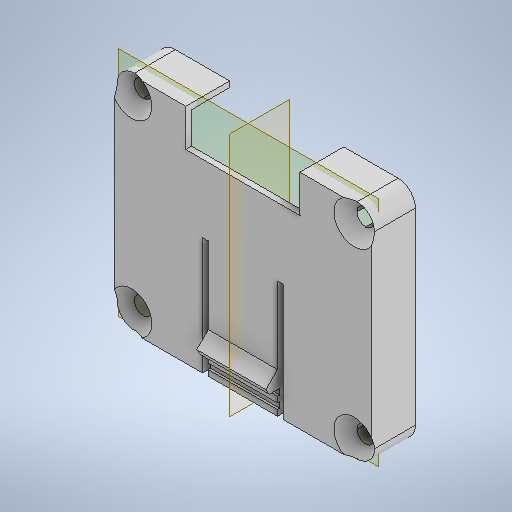
# Autodesk Inventor part: akkum_cap_pd
Saved by Autodesk Inventor 2025 (Build 290162000, 162)
## iProperties
Created: 2026-06-28
Part Number: akkum_cap_pd
Material: Типовые
Document SubType Name: Modeling
Designer: garin
Density: 1 g/cm^3
Appearance: По умолчанию
Author: garin
Autodesk Inventor part; units mm, degrees
ref_plane "YZ Plane" through (0, 0, 0) normal (1, 0, 0) x (0, 1, 0)
ref_plane "XZ Plane" through (0, 0, 0) normal (0, 1, 0) x (-1, 0, 0)
ref_plane "XY Plane" through (0, 0, 0) normal (0, 0, 1) x (1, 0, 0)
sketch "Эскиз1" plane through (0, 0, 0) normal (0, 0, 1) x (1, 0, 0)
  arc A0 (-22.3, -16.3) -> (-19.3, -19.3) centre (-19.3, -16.3) ccw
  line L0 (-22.3, -16.3) -> (-22.3, 16.3)
  arc A1 (-19.3, 19.3) -> (-22.3, 16.3) centre (-19.3, 16.3) ccw
  line L1 (-19.3, 19.3) -> (19.3, 19.3)
  arc A2 (22.3, 16.3) -> (19.3, 19.3) centre (19.3, 16.3) ccw
  line L2 (22.3, 16.3) -> (22.3, -16.3)
  arc A3 (19.3, -19.3) -> (22.3, -16.3) centre (19.3, -16.3) ccw
  line L3 (19.3, -19.3) -> (-19.3, -19.3)
  circle A4 centre (19.3, 16.3) radius 2 construction
  circle A5 centre (-19.3, 16.3) radius 2 construction
  circle A6 centre (-19.3, -16.3) radius 2 construction
  circle A7 centre (19.3, -16.3) radius 2 construction
  arc A8 (-1.4869, 14.15) -> (-14.15, 1.4869) centre (-9.15, 9.15) ccw
  line L4 (-14.15, 1.4869) -> (-14.15, -1.4869)
  arc A9 (-14.15, -1.4869) -> (-1.4869, -14.15) centre (-9.15, -9.15) ccw
  line L5 (-1.4869, -14.15) -> (1.4869, -14.15)
  arc A10 (1.4869, -14.15) -> (14.15, -1.4869) centre (9.15, -9.15) ccw
  line L6 (14.15, -1.4869) -> (14.15, 1.4869)
  arc A11 (14.15, 1.4869) -> (1.4869, 14.15) centre (9.15, 9.15) ccw
  line L7 (1.4869, 14.15) -> (-1.4869, 14.15)
  line L8 (-9.15, 9.15) -> (-9.15, 18.3) construction
  line L9 (9.15, 9.15) -> (9.15, 18.3) construction
  line L10 (-9.15, 9.15) -> (-18.3, 9.15) construction
  line L11 (-9.15, -9.15) -> (-18.3, -9.15) construction
  line L12 (-18.3, 9.15) -> (-18.3, -9.15)
  line L13 (-9.15, 18.3) -> (9.15, 18.3)
  line L14 (-22.3, 0) -> (22.3, 0) construction
  line L15 (0, 19.3) -> (0, -19.3) construction
  line L16 (18.3, 9.15) -> (18.3, -9.15)
  line L17 (-9.15, -18.3) -> (9.15, -18.3)
  circle A12 centre (-19.3, 16.3) radius 1.5
  circle A13 centre (19.3, 16.3) radius 1.5
  circle A14 centre (19.3, -16.3) radius 1.5
  circle A15 centre (-19.3, -16.3) radius 1.5
  line L18 (0, 19.3) -> (-9.9, 19.3) construction
  line L19 (-9.9, 19.3) -> (-9.9, 12.8) construction
  line L20 (-9.9, 12.8) -> (0, 12.8) construction
  line L21 (0, 12.8) -> (0, 19.3) construction
  line L22 (-9.9, 12.8) -> (9.9, 12.8)
  line L23 (9.9, 12.8) -> (9.9, 19.3)
  line L24 (9.9, 19.3) -> (-9.9, 19.3)
  line L25 (-9.9, 19.3) -> (-9.9, 12.8)
  line L26 (-18.3, 9.15) -> (-18.3, 4.15) construction
  line L27 (-18.3, -9.15) -> (-18.3, -4.15) construction
  line L28 (-18.3, -4.15) -> (-21.5, -4.15)
  line L29 (-21.5, -4.15) -> (-21.5, 4.15)
  line L30 (-21.5, 4.15) -> (-18.3, 4.15)
  line L31 (-18.3, 4.15) -> (-18.3, -4.15)
  line L32 (18.3, -4.15) -> (21.5, -4.15)
  line L33 (21.5, -4.15) -> (21.5, 4.15)
  line L34 (21.5, 4.15) -> (18.3, 4.15)
  line L35 (18.3, 4.15) -> (18.3, -4.15)
  line L36 (-21.5, 0) -> (-21.5, 12.8)
  line L37 (-21.5, 12.8) -> (-17.5405, 12.8)
  line L38 (-21.5, 0) -> (-21.5, -12.8)
  line L39 (-21.5, -12.8) -> (-17.5405, -12.8)
  line L40 (19.3, 14.8) -> (22.3, 14.8)
  line L41 (17.8, 16.3) -> (17.8, 19.3)
  line L42 (-19.3, 14.8) -> (-22.3, 14.8)
  line L43 (-17.8, 16.3) -> (-17.8, 19.3)
  line L44 (17.8, -16.3) -> (17.8, -19.3)
  line L45 (19.3, -14.8) -> (22.3, -14.8)
  line L46 (-17.8, -16.3) -> (-17.8, -19.3)
  line L47 (-19.3, -14.8) -> (-22.3, -14.8)
  line L48 (9.15, 18.3) -> (17.8, 18.3)
  line L49 (-9.15, -18.3) -> (-17.8, -18.3)
  line L50 (9.15, -18.3) -> (17.8, -18.3)
  line L51 (-9.15, 18.3) -> (-17.8, 18.3)
  line L52 (18.3, 4.15) -> (19.3, 4.15)
  line L53 (19.3, 4.15) -> (19.3, 14.8)
  line L54 (19.3, 4.15) -> (19.3, -14.8)
  line L55 (19.3, 4.15) -> (38.25, 4.15) construction
  line L56 (-21.5, 12.8) -> (-21.5, 14.8)
  line L57 (-21.5, -12.8) -> (-21.5, -14.8)
  point P0 (-9.9, 19.3)
  point P1 (9.9, 19.3)
  point P2 (9.9, 18.2692)
  point P3 (-9.9, 18.2692)
  point P4 (19.3, -4.15)
  dimension "d5" = 3
  dimension "d6" = 3
  dimension "d7" = 3
  dimension "d8" = 3
  dimension "d9" = 9.9
  dimension "d10" = 6.5
  dimension "d11" = 19.8
  dimension "d12" = 6.5
  dimension "d13" = 5
  dimension "d14" = 5
  dimension "d15" = 3.2
  dimension "d16" = 8.3
  dimension "d19" = 12.8
  dimension "d51" = 1
  dimension "d52" = 90
  constraints: 116 end point, 32 point on circle, 29 point on line, 16 centre point, 14 perpendicular, 10 symmetric about line, 9 horizontal, 8 parallel, 8 tangent, 6 vertical, 5 midpoint, 4 coincident, 40 other
  measures "d5" diameter of A12
  measures "d6" diameter of A13
  measures "d7" diameter of A14
  measures "d8" diameter of A15
  measures "d9" distance of L20.end L19.end
  measures "d10" distance of L19.end L18.end
  measures "d11" distance of L24.end L23.end
  measures "d12" distance of L23.end L22.end
  measures "d13" distance of L10.end L26.end
  measures "d14" distance of L11.end L27.end
  measures "d15" distance of L29.end L30.end
  measures "d16" distance of L28.end L29.end
  measures "d19" distance of L36.start L36.end
  measures "d51" distance of L35.start L52.end
  measures "d52" angle of L54 L55
extrude "Выдавливание1" add sketch "Эскиз1" along normal blind 7.6 contours L0 L47 A15 L46 L3 A0 | L0 L42 L56 L36 L29 L38 L57 L47 | L46 L49 L17 L50 L44 L3 | L0 A1 L1 L43 A12 L42 | L57 L39 A9 L49 L46 A15 L47 | L44 A14 L45 L2 A3 L3 | L42 A12 L43 L51 L25 A8 L37 L56 | L38 L28 L12 A9 L39 | L50 A10 L16 L32 L54 A14 L44 | A9 L4 A8 L25 L22 L23 A11 L6 A10 L5 | A9 L5 A10 L17 | L37 A8 L12 L30 L36 | L29 L30 L12 L28 | L1 L25 L51 L43 | L12 A8 L4 A9 | L45 L54 L32 L33 L34 L53 L40 L2 | A10 L6 A11 L16 | L40 A13 L41 L1 A2 L2 | L54 L34 L33 L32 | L32 L16 L34 L54 | L1 L41 L48 L23 | L53 L34 L16 A11 L23 L48 L41 A13
chamfer "Фаска1" distance 2 angle 45 4 edges at (17.8, 16.3, 7.6) (-20.8, 16.3, 7.6) (-20.8, -16.3, 7.6) (17.8, -16.3, 7.6)
extrude "Выдавливание2" cut sketch "Эскиз1" along normal blind 6.6 contours L38 L28 L12 A9 L39 | A9 L4 A8 L25 L22 L23 A11 L6 A10 L5 | A9 L5 A10 L17 | L37 A8 L12 L30 L36 | L29 L30 L12 L28 | L12 A8 L4 A9 | A10 L6 A11 L16 | L54 L34 L33 L32 | L32 L16 L34 L54
sketch "Эскиз2" plane through (-22.3, -16.3, 0) normal (-1, 0, 0) x (0, 0, 1)
  line L0 (0, -3) -> (0, 0) projected
  line L1 (0, 35.6) -> (7.1, 35.6) projected
  line L2 (0, -3) -> (0, 35.6) construction
  line L3 (0, 16.3) -> (7.6, 16.3) construction
  line L4 (7.6, 30.7972) -> (7.6, 1.8028) projected
  line L5 (0, 16.3) -> (1, 16.3) construction
  line L6 (1, 16.3) -> (1, 20.5) construction
  line L7 (1, 20.5) -> (0, 20.5) construction
  line L8 (0, 20.5) -> (0, 16.3) construction
  line L9 (1, 20.5) -> (3.6, 20.5)
  line L10 (3.6, 20.5) -> (3.6, 12.1)
  line L11 (3.6, 12.1) -> (1, 12.1)
  line L12 (1, 12.1) -> (1, 20.5)
  line L13 (1, 20.5) -> (2.3, 20.5) construction
  line L14 (2.3, 20.5) -> (2.3, 19.2) construction
  line L15 (2.3, 19.2) -> (1, 19.2) construction
  line L16 (1, 19.2) -> (1, 20.5) construction
  arc A0 (3.6, 19.2) -> (1, 19.2) centre (2.3, 19.2) ccw
  arc A1 (1, 13.4) -> (3.6, 13.4) centre (2.3, 13.4) ccw
  point P0 (3.6, 13.4)
  point P1 (1, 19.2)
  point P2 (1, 13.4)
  point P3 (2.3, 12.1)
  point P4 (2.3, 20.5)
  dimension "d20" = 1
  dimension "d21" = 4.2
  dimension "d22" = 2.6
  dimension "d23" = 8.4
  dimension "d24" = 1.3
  dimension "d25" = 1.3
  constraints: 28 end point, 6 parallel, 5 point on circle, 3 horizontal, 3 perpendicular, 3 symmetric about line, 2 centre point, 2 point on line, 1 midpoint, 1 vertical, 1 other
  measures "d20" distance of L7.end L6.end
  measures "d21" distance of L6.end L5.end
  measures "d22" distance of L10.end L11.end
  measures "d23" distance of L9.end L10.end
  measures "d24" distance of L14.end L15.end
  measures "d25" distance of L13.end L14.end
extrude "Выдавливание3" cut sketch "Эскиз2" against normal blind 0.8 contours A0 L10 A1 L12
fillet "Сопряжение1" radius 2 1 edges at (21.5, 0, 6.6)
sketch "Эскиз3" plane through (0, 0, 7.6) normal (0, 0, 1) x (1, 0, 0)
  line L0 (-19.3, -19.3) -> (19.3, -19.3) projected
  line L1 (0, -19.3) -> (-6, -19.3)
  line L2 (-6, -19.3) -> (6, -19.3)
  line L3 (6, -19.3) -> (6, 0)
  line L4 (6, 0) -> (-6, 0)
  line L5 (-6, 0) -> (-6, -19.3)
  line L6 (-7, 1) -> (7, 1)
  line L7 (7, 1) -> (7, -20.3)
  line L8 (7, -20.3) -> (-7, -20.3)
  line L9 (-7, -20.3) -> (-7, 1)
  line L10 (-6, -19.3) -> (6, -19.3)
  line L11 (6, -19.3) -> (6, -17.3)
  line L12 (6, -17.3) -> (-6, -17.3)
  line L13 (-6, -17.3) -> (-6, -19.3)
  line L14 (-6, 0) -> (-6, 1)
  line L15 (6, 0) -> (6, 1)
  line L16 (-6, -17.3) -> (6, -17.3)
  line L17 (6, -17.3) -> (6, -18.3)
  line L18 (6, -18.3) -> (-6, -18.3)
  line L19 (-6, -18.3) -> (-6, -17.3)
  line L20 (-6, -17.3) -> (6, -17.3)
  line L21 (6, -17.3) -> (6, -16.3)
  line L22 (6, -16.3) -> (-6, -16.3)
  line L23 (-6, -16.3) -> (-6, -17.3)
  line L24 (-6, -16.3) -> (6, -16.3)
  line L25 (6, -16.3) -> (6, -15.3)
  line L26 (6, -15.3) -> (-6, -15.3)
  line L27 (-6, -15.3) -> (-6, -16.3)
  point P0 (0, 0)
  point P1 (7, -19.3)
  point P2 (-7, -19.3)
  dimension "d29" = 6
  dimension "d30" = 12
  dimension "d31" = 19.3
  dimension "d32" = 1
  dimension "d33" = 2
  dimension "d40" = 1
  dimension "d43" = 1
  constraints: 54 end point, 12 parallel, 8 perpendicular, 6 point on line, 5 horizontal, 2 midpoint, 3 other
  measures "d29" distance of L1.start L1.end
  measures "d30" distance of L4.end L3.end
  measures "d31" distance of L3.end L2.end
  measures "d32" distance between parallel lines of L4 L6
  measures "d33" distance of L11.end L10.end
  measures "d40" distance of L21.end L20.end
  measures "d43" distance of L25.end L24.end
extrude "Выдавливание4" cut sketch "Эскиз3" against normal blind 10 contours L0 L9 L6 L14 L5 | L3 L15 L6 L7 L0
sketch "Эскиз5" plane through (-6, -19.3, 0) normal (0, -1, 0) x (1, 0, 0)
  line L0 (0, 0) -> (12, 0) projected
  line L1 (0, 0) -> (12, 0)
  line L2 (12, 0) -> (12, 5.4)
  line L3 (12, 5.4) -> (0, 5.4)
  line L4 (0, 5.4) -> (0, 0)
  point P0 (6, 0)
  dimension "d36" = 12
  dimension "d37" = 5.4
  constraints: 8 end point, 2 parallel, 1 horizontal, 1 perpendicular
  measures "d36" distance of L3.end L2.end
  measures "d37" distance of L2.end L1.end
extrude "Выдавливание5" cut sketch "Эскиз5" against normal blind 10
extrude "Выдавливание6" cut sketch "Эскиз3" against normal blind 0.4 contours L5 L12 L3 L18 | L5 L26 L3 L22
sketch "Эскиз6" plane through (6, -18.3, 6.6) normal (1, 0, 0) x (0, 0, -1)
  line L0 (-1, 19.3) -> (-1, 3) projected
  line L1 (-1, 3) -> (-4, 3)
  line L2 (-4, 3) -> (-1, 6)
  line L3 (-4, 3) -> (0.2426, 3) construction
  line L4 (-1, 6) -> (-1, 3)
  line L5 (-1, 3) -> (-3, 3)
  line L6 (-3, 3) -> (-3, 4)
  line L7 (-3, 4) -> (-1, 4)
  line L8 (-1, 4) -> (-1, 3)
  line L9 (-3, 4) -> (-2.4226, 3)
  line L10 (-3, 4) -> (-1.8453, 4) construction
  point P0 (6.6, 18.3)
  point P1 (-3, 3)
  point P2 (-2.4226, 3)
  dimension "d44" = 3
  dimension "d48" = 45
  dimension "d49" = 2
  dimension "d50" = 60
  constraints: 20 end point, 4 horizontal, 3 point on line, 2 equal length, 2 parallel, 1 perpendicular, 1 vertical
  measures "d44" distance of L0.end L1.end
  measures "d48" angle of L3 L2
  measures "d49" distance of L6.end L7.end
  measures "d50" angle of L9 L10
extrude "Выдавливание7" add sketch "Эскиз6" against normal blind 12 contours L0 L7 L2 | L0 L1 L9 L7
ref_plane "РабПлоскость1" through (0, -16.3, 0) normal (1, 0, 0) x (0, 0, -1)
sketch "Эскиз9" plane through (0, -16.3, 0) normal (1, 0, 0) x (0, 0, -1)
  point P0 (0, 16.3)
ref_plane "РабПлоскость2" through (0, 0, 5.6) normal (0, 0, -1) x (-1, 0, 0)
extrude "Выдавливание8" cut sketch "Эскиз1" against normal blind 5.6 from surface at 5.6 contours L57 L39 A9 L49 L46 A15 L47 | L42 A12 L43 L51 L25 A8 L37 L56 | L50 A10 L16 L32 L54 A14 L44 | L25 L51 A8 | L53 L34 L16 A11 L23 L48 L41 A13 | L23 A11 L48
